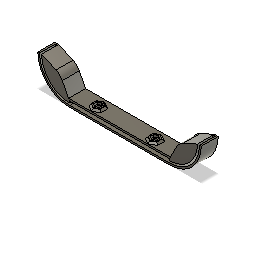
Metal Plus Feet (Autodesk Fusion 360 design; units mm, degrees)
Autodesk Fusion 360 part; units mm, degrees
sketch "Sketch1" plane through (-12.1056, -310.0221, -84.0621) normal (0, 0, -1) x (1, 0, 0)
  line L0 (-44.45, 0.8001) -> (44.45, 0.8001)
  line L1 (42.8498, -2.319) -> (-42.8498, -2.319)
  arc A0 (-44.45, 0.8001) -> (-71.4502, -26.2001) centre (-44.45, -26.2001) ccw
  arc A1 (71.4502, -26.2001) -> (44.45, 0.8001) centre (44.45, -26.2001) ccw
  arc A2 (-44.45, -0.8001) -> (-69.85, -26.2001) centre (-44.45, -26.2001) ccw
  arc A3 (69.85, -26.2001) -> (44.45, -0.8001) centre (44.45, -26.2001) ccw
  arc A4 (71.5502, -26.2001) -> (44.45, 0.9001) centre (44.45, -26.2001) ccw
  line L2 (-44.45, 0.9001) -> (44.45, 0.9001)
  arc A5 (-44.45, 0.9001) -> (-71.5502, -26.2001) centre (-44.45, -26.2001) ccw
  arc A6 (69.75, -26.2001) -> (44.7498, -0.9019) centre (44.45, -26.2001) ccw
  line L3 (42.8498, -2.419) -> (-42.8498, -2.419)
  arc A7 (-44.7498, -0.9019) -> (-69.75, -26.2001) centre (-44.45, -26.2001) ccw
  line L4 (-42.8498, -2.419) -> (-44.7498, -2.419)
  line L5 (-44.7498, -2.419) -> (-44.7498, -0.9019)
  line L6 (0, 0) -> (0, 7.9071) construction
  line L7 (44.7498, -2.419) -> (44.7498, -0.9019)
  line L8 (42.8498, -2.419) -> (44.7498, -2.419)
  line L9 (71.5502, -26.2001) -> (69.75, -26.2001)
  line L10 (-71.5502, -26.2001) -> (-69.75, -26.2001)
  line L11 (-69.75, -26.2001) -> (-56.9141, -20.3456)
  line L12 (-44.7498, -2.419) -> (-51.2381, -14.9465)
  arc A8 (-56.9141, -20.3456) -> (-51.2381, -14.9465) centre (-61.8938, -9.4276) ccw
  line L13 (44.7498, -2.419) -> (51.2381, -14.9465)
  arc A9 (51.2381, -14.9465) -> (56.9141, -20.3456) centre (61.8938, -9.4276) ccw
  line L14 (69.75, -26.2001) -> (56.9141, -20.3456)
  line L15 (-45.5785, -4.019) -> (45.5785, -4.019)
  arc A10 (73.1502, -26.2001) -> (44.45, 2.5001) centre (44.45, -26.2001) ccw
  line L16 (-44.45, 2.5001) -> (44.45, 2.5001)
  arc A11 (-44.45, 2.5001) -> (-73.1502, -26.2001) centre (-44.45, -26.2001) ccw
  line L17 (-73.1502, -26.2001) -> (-71.5502, -26.2001)
  line L18 (73.1502, -26.2001) -> (71.5502, -26.2001)
  dimension "d522" = 1.9
  dimension "d523" = 12
  dimension "d524" = 1.6
  dimension "d525" = 1.7
  constraint parallel L3 L4
  constraint perpendicular L4 L5
  constraint concentric A2 A7
  constraint coincident L6.start origin
  constraint perpendicular L0 L6
  constraint symmetric L3.end L6 L3.start
  constraint symmetric L4.end L6 L7.start
  constraint symmetric A7.start L6 A6.end
  constraint concentric A3 A6
  constraint horizontal L9
  constraint symmetric A4.start L6 A5.end
  constraint symmetric A6.start L6 A7.end
  constraint tangent L11 A8
  constraint tangent L12 A8
  constraint symmetric A7.end L6 A6.start
  constraint symmetric L6 L11.end A9.end
  constraint symmetric L6 L12.end L13.end
  constraint symmetric L6 A8 A9
  constraint coincident L12 L15.start
  constraint coincident L13 L15.end
  constraint parallel L3 L15
  constraint parallel L10 L17
  constraint parallel L15 L18
  measures "d522" distance of L3.end L4.end
  measures "d523" radius of A8
  measures "d524" distance of L3 L15
extrude "Extrude1" add sketch "Sketch1" against normal blind 14 contours A4 L2 A5 A10 L16 A11 L17 L18 | A7 L5 L11 L12 A8 | A6 L7 L13 A9 L14 | L3 L4 L8 L12 L13 L15 makes body 1 at (-26.9222, -312.5222, -79.3954) makes body 2 at (-27.2984, -306.0031, -79.3954)
extrude "Extrude2" add sketch "Sketch1" along normal blind 1.2 bodies 1 2
sketch "Sketch2" plane through (0, -312.5222, 0) normal (0, -1, 0) x (1, 0, 0)
  line L0 (32.3444, -85.2621) -> (32.3444, -70.0621)
  line L1 (32.3444, -70.0621) -> (-56.5556, -70.0621)
  line L2 (-56.5556, -70.0621) -> (-56.5556, -85.2621)
  line L3 (-56.5556, -85.2621) -> (32.3444, -85.2621)
  circle A0 centre (-37.5056, -76.4421) radius 1.75
  circle A1 centre (13.2944, -76.4421) radius 1.75
  circle A2 centre (-37.5056, -76.4421) radius 1.5
  circle A3 centre (13.2944, -76.4421) radius 1.5
  dimension "d530" = 3
  dimension "d531" = 3
  constraint concentric A0 A2
  constraint concentric A1 A3
  measures "d530" diameter of A2
  measures "d531" diameter of A3
extrude "Extrude3" cut sketch "Sketch2" against normal blind 1.6 contours A2 | A3 bodies 1
sketch "Sketch3" plane through (0, -307.6031, 0) normal (0, -1, 0) x (1, 0, 0)
  line L0 (-56.8554, -84.0621) -> (32.6442, -84.0621)
  line L1 (32.6442, -84.0621) -> (32.6442, -70.0621)
  line L2 (32.6442, -70.0621) -> (-56.8554, -70.0621)
  line L3 (-56.8554, -70.0621) -> (-56.8554, -84.0621)
  circle A0 centre (-37.5056, -76.4421) radius 1.5
  circle A1 centre (13.2944, -76.4421) radius 1.5
  circle A2 centre (-37.5056, -76.4421) radius 1.6
  circle A3 centre (13.2944, -76.4421) radius 1.6
  dimension "d534" = 3.2
  dimension "d535" = 3.2
  constraint concentric A0 A2
  constraint concentric A1 A3
  measures "d534" diameter of A2
  measures "d535" diameter of A3
extrude "Extrude4" cut sketch "Sketch3" against normal blind 5 contours A0 | A1 | A2 | A3 bodies 1
sketch "Sketch4" plane through (0, -306.0031, 0) normal (0, 1, 0) x (-1, 0, 0)
  circle A0 centre (37.5056, -76.4421) radius 1.6
  circle A1 centre (-13.2944, -76.4421) radius 1.6
  line L0 (-33.4729, -70.0621) -> (-33.4729, -85.2621)
  line L1 (-33.4729, -85.2621) -> (57.6841, -85.2621)
  line L2 (57.6841, -85.2621) -> (57.6841, -70.0621)
  line L3 (57.6841, -70.0621) -> (-33.4729, -70.0621)
  line L4 (-10.5944, -74.8832) -> (-13.2944, -73.3244)
  line L5 (-13.2944, -73.3244) -> (-15.9944, -74.8832)
  line L6 (-15.9944, -74.8832) -> (-15.9944, -78.0009)
  line L7 (-15.9944, -78.0009) -> (-13.2944, -79.5598)
  line L8 (-13.2944, -79.5598) -> (-10.5944, -78.0009)
  line L9 (-10.5944, -78.0009) -> (-10.5944, -74.8832)
  line L10 (-13.2944, -76.4421) -> (37.5056, -76.4421) construction
  line L11 (12.1056, -76.4421) -> (12.1056, -73.2007) construction
  line L12 (34.8056, -74.8832) -> (37.5056, -73.3244)
  line L13 (37.5056, -73.3244) -> (40.2056, -74.8832)
  line L14 (40.2056, -74.8832) -> (40.2056, -78.0009)
  line L15 (40.2056, -78.0009) -> (37.5056, -79.5598)
  line L16 (37.5056, -79.5598) -> (34.8056, -78.0009)
  line L17 (34.8056, -78.0009) -> (34.8056, -74.8832)
  line L18 (-17.1944, -74.1904) -> (-17.1944, -78.6937)
  line L19 (-17.1944, -78.6937) -> (-13.2944, -80.9454)
  line L20 (-13.2944, -80.9454) -> (-9.3944, -78.6937)
  line L21 (-9.3944, -78.6937) -> (-9.3944, -74.1904)
  line L22 (-9.3944, -74.1904) -> (-13.2944, -71.9387)
  line L23 (-13.2944, -71.9387) -> (-17.1944, -74.1904)
  line L24 (37.5056, -71.9387) -> (41.4056, -74.1904)
  line L25 (33.6056, -74.1904) -> (37.5056, -71.9387)
  line L26 (33.6056, -78.6937) -> (33.6056, -74.1904)
  line L27 (37.5056, -80.9454) -> (33.6056, -78.6937)
  line L28 (41.4056, -78.6937) -> (37.5056, -80.9454)
  line L29 (41.4056, -74.1904) -> (41.4056, -78.6937)
  point P0 (-13.2944, -76.4421)
  dimension "d538" = 2.7
  dimension "d539" = 1.2
  constraint coincident P0 A1.centre
  constraint coincident A0.centre L10.end
  constraint midpoint L10 L11.start
  constraint perpendicular L10 L11
  constraint symmetric L4.start L11 L12.start
  constraint symmetric L4.end L11 L12.end
  constraint symmetric L5.end L11 L13.end
  constraint symmetric L6.end L11 L14.end
  constraint symmetric L7.end L11 L15.end
  constraint symmetric L8.end L11 L16.end
  constraint symmetric L11 L18.start L24.end
  constraint symmetric L11 L18.end L28.start
  constraint symmetric L11 L19.end L27.start
  constraint symmetric L11 L20.end L26.start
  constraint symmetric L11 L21.end L25.start
  constraint symmetric L11 L22.end L24.start
  measures "d538" distance of P0 L9
extrude "Extrude6" add sketch "Sketch4" along normal blind 2 contours L18 L19 L20 L21 L22 L23 | L24 L25 L26 L27 L28 L29 bodies 1
chamfer "Chamfer2" distance 1.5 angle 45 12 edges at (-39.4556, -306.0031, -79.8196) (-41.4056, -306.0031, -76.4421) (-33.6056, -306.0031, -76.4421) (15.2444, -306.0031, -79.8196) (17.1944, -306.0031, -76.4421) (9.3944, -306.0031, -76.4421) (11.3444, -306.0031, -73.0646) (15.2444, -306.0031, -73.0646) (-35.5556, -306.0031, -73.0646) (-39.4556, -306.0031, -73.0646) (-35.5556, -306.0031, -79.8196) (11.3444, -306.0031, -79.8196) on bodies 1
extrude "Extrude5" [suppressed]
chamfer "Chamfer1" [suppressed]
equation "d517 = -foff"
equation "d519 = -foff"
equation "d525 = 1.6 mm + foff"
equation "d538 = ( 5.4 / 2 ) * 1 mm"
equation "foff = 0.1 mm" comment "tolerance offset between feet and case"
